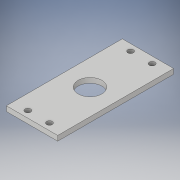
# Autodesk Inventor part: came1
Saved by Autodesk Inventor 2019 (Build 230136000, 136)
## iProperties
Created: 2021-11-17
Part Number: came1
Material: 一般
Document SubType Name: Modeling
Designer: yuta
Density: 1 g/cm^3
Appearance: 既定
Author: yuta
Autodesk Inventor part; units mm, degrees
ref_plane "YZ Plane" through (0, 0, 0) normal (1, 0, 0) x (0, 1, 0)
ref_plane "XZ Plane" through (0, 0, 0) normal (0, 1, 0) x (-1, 0, 0)
ref_plane "XY Plane" through (0, 0, 0) normal (0, 0, 1) x (1, 0, 0)
sketch "スケッチ1" plane through (0, 0, 0) normal (0, 1, 0) x (-1, 0, 0)
  line L0 (4.9789, 14.724) -> (-26.0211, 14.724)
  line L1 (-26.0211, 14.724) -> (-26.0211, -55.276)
  line L2 (-26.0211, -55.276) -> (4.9789, -55.276)
  line L3 (4.9789, -55.276) -> (4.9789, 14.724)
  point P0 (0, 0)
  dimension "d0" = 31
  dimension "d1" = 70
  constraints: 8 end point, 2 parallel, 1 horizontal, 1 perpendicular
  measures "d0" distance of L2.end L1.end
  measures "d1" distance of L1.end L0.end
extrude "押し出し1" add sketch "スケッチ1" along normal blind 3
sketch "スケッチ2" plane through (0, 3, 0) normal (0, 1, 0) x (1, 0, 0)
  circle A0 centre (4.0211, -10.724) radius 1.7
  circle A1 centre (17.0211, -10.724) radius 1.7
  line L0 (-4.9789, 55.276) -> (-4.9789, -14.724) projected
  line L1 (26.0211, -14.724) -> (26.0211, 55.276) projected
  line L2 (-4.9789, -14.724) -> (26.0211, -14.724) projected
  circle A2 centre (4.0211, 51.276) radius 1.7
  line L3 (26.0211, 55.276) -> (-4.9789, 55.276) projected
  circle A3 centre (17.0211, 51.276) radius 1.7
  circle A4 centre (10.5211, 20.276) radius 7.15
  point P0 (0, 0)
  dimension "d4" = 3.4
  dimension "d5" = 3.4
  dimension "d6" = 9
  dimension "d7" = 9
  dimension "d8" = 4
  dimension "d9" = 4
  dimension "d10" = 3.4
  dimension "d11" = 9
  dimension "d12" = 4
  dimension "d13" = 3.4
  dimension "d14" = 9
  dimension "d15" = 4
  dimension "d16" = 14.3
  dimension "d17" = 35
  dimension "d18" = 15.5
  constraints: 5 centre point
  measures "d4" diameter of A0
  measures "d5" diameter of A1
  measures "d6" distance from line of L0 A0.centre
  measures "d7" distance from line of L1 A1.centre
  measures "d8" distance from line of L2 A0.centre
  measures "d9" distance from line of L2 A1.centre
  measures "d10" diameter of A2
  measures "d11" distance from line of L0 A2.centre
  measures "d12" distance from line of L3 A2.centre
  measures "d13" diameter of A3
  measures "d14" distance from line of L1 A3.centre
  measures "d15" distance from line of L3 A3.centre
  measures "d16" diameter of A4
  measures "d17" distance from line of L3 A4.centre
  measures "d18" distance from line of L0 A4.centre
hole "穴1" at (4.0211, 3, 10.724) at (17.0211, 3, 10.724) at (17.0211, 3, -51.276) at (4.0211, 3, -51.276) direction (0, -1, 0) diameter 3.4 depth 3
sketch "スケッチ3" plane through (0, 3, 0) normal (0, 1, 0) x (1, 0, 0)
  circle A0 centre (10.5211, 20.276) radius 7.15
  line L0 (-4.9789, 55.276) -> (-4.9789, -14.724) projected
  line L1 (-4.9789, -14.724) -> (26.0211, -14.724) projected
  point P0 (0, 0)
  dimension "d26" = 14.3
  dimension "d27" = 15.5
  dimension "d28" = 35
  constraints: 1 centre point
  measures "d26" diameter of A0
  measures "d27" distance from line of L0 A0.centre
  measures "d28" distance from line of L1 A0.centre
extrude "押し出し2" cut sketch "スケッチ3" against normal blind 3
